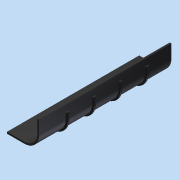
# Autodesk Inventor part: Grip
Saved by Autodesk Inventor 2011 SP1 (Build 150282100, 282)
## iProperties
Created: 2011-08-16
Part Number: Grip
Document SubType Name: Modeling
Designer: dgitz
Density: 1 g/cm^3
Author: dgitz
Autodesk Inventor part; units mm, degrees
ref_plane "YZ Plane" through (0, 0, 0) normal (1, 0, 0) x (0, 1, 0)
ref_plane "XZ Plane" through (0, 0, 0) normal (0, 1, 0) x (-1, 0, 0)
sketch "Sketch1" plane through (0, 0, 0) normal (0, 0, 1) x (1, 0, 0)
  line L0 (-2.4289, 0) -> (-2.4289, 12.7)
  line L1 (-2.4289, 12.7) -> (-4.0164, 12.7)
  line L2 (-4.0164, 12.7) -> (-4.0164, 0)
  line L3 (-4.0164, 0) -> (-29.4164, 0) construction
  line L4 (-33.2939, -14.2875) -> (-33.2939, -12.7)
  line L5 (-33.2939, -12.7) -> (-16.7164, -12.7)
  line L6 (-16.7164, -14.2875) -> (-33.2939, -14.2875)
  arc A0 (-16.7164, -14.2875) -> (-2.4289, 0) centre (-16.7164, 0) ccw
  arc A1 (-16.7164, -12.7) -> (-4.0164, 0) centre (-16.7164, 0) ccw
  dimension "d5" = 1.5875
  dimension "d9" = 1.5875
  constraints: 14 end point, 4 point on circle, 2 centre point, 1 coincident, 1 midpoint, 1 parallel, 1 perpendicular, 1 vertical
  measures "d5" distance of L0.end L1.end
  measures "d9" distance of L4.start L4.end
extrude "Extrusion1" add sketch "Sketch1" along normal blind 127
ref_plane "Work Plane1" through (0, 0, 101.6) normal (0, 0, 1) x (1, 0, 0)
sketch "Sketch2" plane through (0, 0, 101.6) normal (0, 0, 1) x (1, 0, 0)
  arc A0 (-16.7164, -14.2875) -> (-2.4289, 0) centre (-16.7164, 0) ccw projected
  arc A1 (-16.7164, -14.2875) -> (-2.4289, 0) centre (-16.7164, 0) ccw
  line L0 (-0.8414, 0) -> (-0.8414, 6.35)
  line L1 (-0.8414, 6.35) -> (-2.4289, 6.35)
  line L2 (-2.4289, 0) -> (-2.4289, 12.7) projected
  line L3 (-16.7164, -15.875) -> (-23.0664, -15.875)
  line L4 (-23.0664, -15.875) -> (-23.0664, -14.2875)
  line L5 (-16.7164, -14.2875) -> (-33.2939, -14.2875) projected
  line L6 (-23.0664, -14.2875) -> (-16.7164, -14.2875)
  line L7 (-2.4289, 6.35) -> (-2.4289, 0)
  arc A2 (-16.7164, -15.875) -> (-0.8414, 0) centre (-16.7164, 0) ccw
  line L8 (-16.7164, 0) -> (-16.7164, -14.2875) construction
  line L9 (-16.7164, -15.875) -> (-16.7164, -20.4579) construction
  point P0 (0, 0)
  dimension "d14" = 6.35
  dimension "d15" = 6.35
  constraints: 16 end point, 6 tangent, 4 point on circle, 2 centre point, 2 coincident, 2 collinear, 2 parallel, 1 midpoint, 1 perpendicular, 1 point on line, 1 vertical
  measures "d14" distance of L0.start L0.end
  measures "d15" distance of L3.start L3.end
extrude "Extrusion2" add sketch "Sketch2" against normal blind 3.175
fillet "Fillet1" radius 1.5875 8 edges at (-0.8414, 6.35, 100.0125) (-5.4911, -11.2253, 101.6) (-0.8414, 3.175, 101.6) (-19.8914, -15.875, 101.6) (-5.4911, -11.2253, 98.425) (-0.8414, 3.175, 98.425) (-19.8914, -15.875, 98.425) (-23.0664, -15.875, 100.0125)
pattern_linear "Rectangular Pattern1" count 4 spacing 25.4 along (0, 0, -1) of "Extrusion2", "Fillet1"
body "Solid1"
